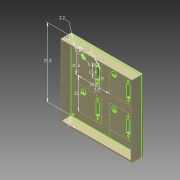
# Autodesk Inventor part: CameraBoardCover2
Saved by Autodesk Inventor 2015 (Build 190159000, 159)
## iProperties
Created: 2015-04-23
Part Number: CameraBoardCover2
Material: NylonD2W
Document SubType Name: Modeling
Designer: Akovo_000
Density: 1.13 g/cm^3
Appearance: Nylon 6
Mass: 18.5115 g
Surface Area: 190.887 cm^2
Volume: 16.3819 cm^3
Author: Akovo_000
Autodesk Inventor part; units mm, degrees
ref_plane "YZ Plane" through (0, 0, 0) normal (1, 0, 0) x (0, 1, 0)
ref_plane "XZ Plane" through (0, 0, 0) normal (0, 1, 0) x (-1, 0, 0)
ref_plane "XY Plane" through (0, 0, 0) normal (0, 0, 1) x (1, 0, 0)
sketch "Sketch1" plane through (0, 0, 0) normal (0, 1, 0) x (-1, 0, 0)
  line L0 (11.1363, 25.3079) -> (-64.3637, 25.3079)
  line L1 (-64.3637, 25.3079) -> (-64.3637, -50.1921)
  line L2 (-64.3637, -50.1921) -> (11.1363, -50.1921)
  line L3 (11.1363, -50.1921) -> (11.1363, 25.3079)
  circle A0 centre (8.9363, 23.1079) radius 1.1
  circle A1 centre (-62.1637, 23.1079) radius 1.1
  circle A2 centre (-62.1637, -47.9921) radius 1.1
  circle A3 centre (8.9363, -47.9921) radius 1.1
  line L4 (8.9363, 23.1079) -> (11.1363, 23.1079) construction
  line L5 (8.9363, 23.1079) -> (8.9363, 25.3079) construction
  line L6 (-62.1637, 25.3079) -> (-62.1637, 23.1079) construction
  line L7 (-62.1637, 23.1079) -> (-64.3637, 23.1079) construction
  line L8 (8.9363, -47.9921) -> (11.1363, -47.9921) construction
  line L9 (8.9363, -47.9921) -> (8.9363, -50.1921) construction
  line L10 (-62.1637, -47.9921) -> (-64.3637, -47.9921) construction
  line L11 (-62.1637, -47.9921) -> (-62.1637, -50.1921) construction
  line L12 (3.0363, 17.2079) -> (-22.5637, 17.2079) construction
  line L13 (-22.5637, 17.2079) -> (-22.5637, -8.3921) construction
  line L14 (-22.5637, -8.3921) -> (3.0363, -8.3921) construction
  line L15 (3.0363, -8.3921) -> (3.0363, 17.2079) construction
  circle A4 centre (-2.4637, 12.8079) radius 2.65
  line L16 (12.6363, 26.8079) -> (-65.8637, 26.8079)
  line L17 (-65.8637, 26.8079) -> (-65.8637, -51.6921)
  line L18 (-65.8637, -51.6921) -> (12.6363, -51.6921)
  line L19 (12.6363, -51.6921) -> (12.6363, 26.8079)
  line L20 (-26.6137, 25.3079) -> (-26.6137, 26.8079) construction
  line L21 (12.6363, -12.4421) -> (11.1363, -12.4421) construction
  line L22 (-16.1637, 11.1079) -> (-19.6637, 11.1079)
  line L23 (-19.6637, 11.1079) -> (-19.6637, -2.2921)
  line L24 (-19.6637, -2.2921) -> (-16.1637, -2.2921)
  line L25 (-16.1637, -2.2921) -> (-16.1637, 11.1079)
  circle A5 centre (-17.9137, -4.7921) radius 0.9
  circle A6 centre (-17.9137, 13.6079) radius 0.9
  line L26 (-17.9137, -4.7921) -> (-17.9137, -2.2921) construction
  line L27 (-17.9137, 13.6079) -> (-17.9137, 11.1079) construction
  line L28 (-17.9137, 13.6079) -> (-17.9137, 17.2079) construction
  line L29 (-17.9137, -4.7921) -> (-17.9137, -8.3921) construction
  line L30 (6.9363, 25.3079) -> (6.9363, 21.1079) construction
  line L31 (6.9363, 21.1079) -> (11.1363, 21.1079) construction
  line L32 (3.0363, -16.4921) -> (-22.5637, -16.4921) construction
  line L33 (-22.5637, -16.4921) -> (-22.5637, -42.0921) construction
  line L34 (-22.5637, -42.0921) -> (3.0363, -42.0921) construction
  line L35 (3.0363, -42.0921) -> (3.0363, -16.4921) construction
  circle A7 centre (-2.4637, -20.8921) radius 2.65
  line L36 (-16.1637, -22.5921) -> (-19.6637, -22.5921)
  line L37 (-19.6637, -22.5921) -> (-19.6637, -35.9921)
  line L38 (-19.6637, -35.9921) -> (-16.1637, -35.9921)
  line L39 (-16.1637, -35.9921) -> (-16.1637, -22.5921)
  circle A8 centre (-17.9137, -38.4921) radius 0.9
  circle A9 centre (-17.9137, -20.0921) radius 0.9
  line L40 (-17.9137, -38.4921) -> (-17.9137, -35.9921) construction
  line L41 (-17.9137, -20.0921) -> (-17.9137, -22.5921) construction
  line L42 (-17.9137, -20.0921) -> (-17.9137, -16.4921) construction
  line L43 (-17.9137, -38.4921) -> (-17.9137, -42.0921) construction
  line L44 (-30.6637, 17.2079) -> (-56.2637, 17.2079) construction
  line L45 (-56.2637, 17.2079) -> (-56.2637, -8.3921) construction
  line L46 (-56.2637, -8.3921) -> (-30.6637, -8.3921) construction
  line L47 (-30.6637, -8.3921) -> (-30.6637, 17.2079) construction
  circle A10 centre (-36.1637, 12.8079) radius 2.65
  line L48 (-49.8637, 11.1079) -> (-53.3637, 11.1079)
  line L49 (-53.3637, 11.1079) -> (-53.3637, -2.2921)
  line L50 (-53.3637, -2.2921) -> (-49.8637, -2.2921)
  line L51 (-49.8637, -2.2921) -> (-49.8637, 11.1079)
  circle A11 centre (-51.6137, -4.7921) radius 0.9
  circle A12 centre (-51.6137, 13.6079) radius 0.9
  line L52 (-51.6137, -4.7921) -> (-51.6137, -2.2921) construction
  line L53 (-51.6137, 13.6079) -> (-51.6137, 11.1079) construction
  line L54 (-51.6137, 13.6079) -> (-51.6137, 17.2079) construction
  line L55 (-51.6137, -4.7921) -> (-51.6137, -8.3921) construction
  line L56 (-30.6637, -16.4921) -> (-56.2637, -16.4921) construction
  line L57 (-56.2637, -16.4921) -> (-56.2637, -42.0921) construction
  line L58 (-56.2637, -42.0921) -> (-30.6637, -42.0921) construction
  line L59 (-30.6637, -42.0921) -> (-30.6637, -16.4921) construction
  circle A13 centre (-36.1637, -20.8921) radius 2.65
  line L60 (-49.8637, -22.5921) -> (-53.3637, -22.5921)
  line L61 (-53.3637, -22.5921) -> (-53.3637, -35.9921)
  line L62 (-53.3637, -35.9921) -> (-49.8637, -35.9921)
  line L63 (-49.8637, -35.9921) -> (-49.8637, -22.5921)
  circle A14 centre (-51.6137, -38.4921) radius 0.9
  circle A15 centre (-51.6137, -20.0921) radius 0.9
  line L64 (-51.6137, -38.4921) -> (-51.6137, -35.9921) construction
  line L65 (-51.6137, -20.0921) -> (-51.6137, -22.5921) construction
  line L66 (-51.6137, -20.0921) -> (-51.6137, -16.4921) construction
  line L67 (-51.6137, -38.4921) -> (-51.6137, -42.0921) construction
  line L68 (-56.2637, 17.2079) -> (-64.3637, 17.2079) construction
  line L69 (3.0363, 17.2079) -> (11.1363, 17.2079) construction
  line L70 (-30.6637, 17.2079) -> (-30.6637, 25.3079) construction
  line L71 (-30.6637, -42.0921) -> (-30.6637, -50.1921) construction
  dimension "d48" = 75.5
  dimension "d49" = 2.2
  dimension "d51" = 2.2
  dimension "d54" = 5.3
  dimension "d55" = 4.4
  dimension "d56" = 5.5
  dimension "d57" = 1.5
  dimension "d58" = 1.8
  dimension "d59" = 2.5
  dimension "d60" = 13.4
  dimension "d61" = 3.5
  dimension "d62" = 2.9
  dimension "d64" = 4.2
  dimension "d67" = 33.7
  dimension "d70" = 33.7
  dimension "d73" = 25.6
  dimension "d74" = 25.6
  constraints: 144 end point, 28 point on line, 19 perpendicular, 16 centre point, 14 equal length, 8 parallel, 6 horizontal, 6 midpoint, 4 equal radius, 2 vertical, 90 other
  measures "d48" distance of L2.end L0.start
  measures "d49" diameter of A0
  measures "d51" distance of L0.start L4.end
  measures "d54" diameter of A4
  measures "d55" distance from line of L12 A4.centre
  measures "d56" distance from line of L15 A4.centre
  measures "d57" horizontal distance of L2.end L18.end
  measures "d58" diameter of A6
  measures "d59" distance of L27.start L27.end
  measures "d60" distance between parallel lines of L24 L22
  measures "d61" distance between parallel lines of L23 L25
  measures "d62" distance between parallel lines of L13 L23
  measures "d64" distance of L0.start L31.end
  measures "d67" distance of L14.end L35.start
  measures "d70" distance of L14.end L47.start
  measures "d73" distance of L14.end L12.start
  measures "d74" distance of L12.end L12.start
extrude "Edges" add sketch "Sketch1" against normal blind 10 contours L19 L18 L17 L16
extrude "Surface" add sketch "Sketch1" along normal blind 2 contours L3 L2 L1 L0 | L19 L18 L17 L16
body "Solid1"
